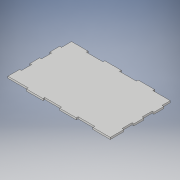
# Autodesk Inventor part: BAWAH
Saved by Autodesk Inventor 2019 (Build 230136000, 136)
## iProperties
Created: 2019-11-24
Part Number: BAWAH
Material: Generic
Document SubType Name: Modeling
Designer: User
Density: 1 g/cm^3
Appearance: Default
Author: User
Autodesk Inventor part; units mm, degrees
ref_plane "YZ Plane" through (0, 0, 0) normal (1, 0, 0) x (0, 1, 0)
ref_plane "XZ Plane" through (0, 0, 0) normal (0, 1, 0) x (-1, 0, 0)
ref_plane "XY Plane" through (0, 0, 0) normal (0, 0, 1) x (1, 0, 0)
sketch "Sketch1" plane through (0, 0, 0) normal (0, 1, 0) x (-1, 0, 0)
  line L0 (55.3, 34) -> (-55.3, -34) construction
  line L1 (-55.3, 34) -> (55.3, -34) construction
  line L2 (35, 34) -> (18.7, 34)
  line L3 (-1.6, 34) -> (-17.9, 34)
  line L4 (35, 34) -> (18.7, 34)
  line L5 (-1.6, 34) -> (-17.9, 34)
  line L6 (-38.2, 34) -> (-53.3, 34)
  line L7 (41.2856, 32.5499) -> (41.2856, 32.5817)
  line L8 (54.8971, 24.1408) -> (54.9227, 24.1408)
  line L9 (-57.3, 34) -> (-55.3, 34)
  line L10 (-57.3, 34) -> (-38.2, 34)
  line L11 (-38.2, 34) -> (-38.2, 32)
  line L12 (-38.2, 32) -> (-19.9, 32)
  line L13 (-19.9, 32) -> (-19.9, 34)
  line L14 (-19.9, 34) -> (-1.6, 34)
  line L15 (-1.6, 34) -> (-1.6, 32)
  line L16 (-1.6, 32) -> (16.7, 32)
  line L17 (16.7, 32) -> (16.7, 34)
  line L18 (16.7, 34) -> (35, 34)
  line L19 (35, 34) -> (35, 32)
  line L20 (35, 32) -> (57.3, 32)
  line L21 (16.7, 34) -> (35, 34)
  line L22 (-55.3, 34) -> (-38.2, 34)
  line L23 (-19.9, 34) -> (-1.6, 34)
  line L24 (-57.3, 34) -> (-57.3, 19)
  line L25 (-57.3, 19) -> (-57.3, 34)
  line L26 (-55.3, -25) -> (-55.3, -34)
  line L27 (-57.3, 19) -> (-55.3, 19)
  line L28 (-55.3, 19) -> (-55.3, 8)
  line L29 (-55.3, 8) -> (-57.3, 8)
  line L30 (-57.3, 8) -> (-57.3, -3)
  line L31 (-57.3, -3) -> (-55.3, -3)
  line L32 (-55.3, -3) -> (-55.3, -14)
  line L33 (-55.3, -14) -> (-57.3, -14)
  line L34 (-57.3, -14) -> (-57.3, -25)
  line L35 (-57.3, -25) -> (-55.3, -25)
  line L36 (-53.3, -34) -> (-55.3, -34)
  line L37 (-53.3, -34) -> (-36.2, -34)
  line L38 (-36.2, -34) -> (-36.2, -36)
  line L39 (-36.2, -36) -> (-17.9, -36)
  line L40 (-17.9, -36) -> (-17.9, -34)
  line L41 (-17.9, -34) -> (0.4, -34)
  line L42 (0.4, -34) -> (0.4, -36)
  line L43 (0.4, -36) -> (18.7, -36)
  line L44 (18.7, -36) -> (18.7, -34)
  line L45 (18.7, -34) -> (37, -34)
  line L46 (37, -34) -> (37, -36)
  line L47 (37, -36) -> (55.3, -36)
  line L48 (55.3, -36) -> (55.3, -25)
  line L49 (55.3, -25) -> (57.3, -25)
  line L50 (57.3, -25) -> (57.3, -14)
  line L51 (57.3, -14) -> (55.3, -14)
  line L52 (55.3, -14) -> (55.3, -3)
  line L53 (55.3, -3) -> (57.3, -3)
  line L54 (57.3, -3) -> (57.3, 8)
  line L55 (57.3, 8) -> (55.3, 8)
  line L56 (55.3, 8) -> (55.3, 19)
  line L57 (55.3, 19) -> (57.3, 19)
  line L58 (57.3, 19) -> (57.3, 32)
  point P0 (-53.3, 32.7703)
  point P1 (1.6, 32)
  point P2 (52.0471, 32)
  point P3 (57.3, -21)
  point P4 (57.3, -35.2297)
  point P5 (57.3, 34)
  point P6 (-57.3, -35.2297)
  point P7 (-55.3, -36)
  dimension "d32" = 19.1
  dimension "d33" = 18.3
  dimension "d34" = 18.3
  dimension "d35" = 18.3
  dimension "d36" = 18.3
  dimension "d53" = 15
  dimension "d54" = 2
  dimension "d55" = 11
  dimension "d56" = 11
  dimension "d58" = 11
  dimension "d59" = 2
  dimension "d60" = 11
  dimension "d62" = 17.1
  dimension "d63" = 18.3
  dimension "d64" = 2
  dimension "d65" = 18.3
  dimension "d66" = 2
  dimension "d67" = 18.3
  dimension "d68" = 2
  dimension "d69" = 18.3
  dimension "d72" = 11
  dimension "d73" = 11
  dimension "d74" = 2
  dimension "d75" = 11
  dimension "d76" = 11
  dimension "d77" = 11
  constraints: 118 end point, 27 perpendicular, 18 point on line, 10 horizontal, 2 vertical, 1 parallel
  measures "d32" distance of L6.start L9.start
  measures "d33" distance of L11.end L12.end
  measures "d34" distance of L3.start L13.end
  measures "d35" distance of L15.end L16.end
  measures "d36" distance of L2.start L17.end
  measures "d53" distance of L9.start L24.end
  measures "d54" distance of L24.end L27.end
  measures "d55" distance of L27.end L28.end
  measures "d56" distance of L29.end L30.end
  measures "d58" distance of L31.end L32.end
  measures "d59" distance of L32.end L33.end
  measures "d60" distance of L33.end L34.end
  measures "d62" distance of L36.start L37.end
  measures "d63" distance of L38.end L39.end
  measures "d64" distance of L39.end L40.end
  measures "d65" distance of L40.end L41.end
  measures "d66" distance of L41.end L42.end
  measures "d67" distance of L42.end L43.end
  measures "d68" distance of L43.end L44.end
  measures "d69" distance of L44.end L45.end
  measures "d72" distance of L47.end L48.end
  measures "d73" distance of L49.end L50.end
  measures "d74" distance of L50.end L51.end
  measures "d75" distance of L51.end L52.end
  measures "d76" distance of L53.end L54.end
  measures "d77" distance of L55.end L56.end
extrude "Extrusion1" add sketch "Sketch1" along normal blind 2
body "Solid1"
